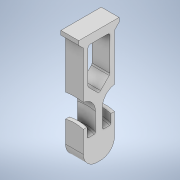
# Autodesk Inventor part: FS-04-SLBV1
Saved by Autodesk Inventor 2022 (Build 260153000, 153)
## iProperties
Created: 2022-01-12
Part Number: FS-04-SLBV1
Material: Generic
Document SubType Name: Modeling
Designer: Frank
Density: 1 g/cm^3
Appearance: Default
Author: Frank
Autodesk Inventor part; units mm, degrees
ref_plane "YZ Plane" through (0, 0, 0) normal (1, 0, 0) x (0, 1, 0)
ref_plane "XZ Plane" through (0, 0, 0) normal (0, 1, 0) x (-1, 0, 0)
ref_plane "XY Plane" through (0, 0, 0) normal (0, 0, 1) x (1, 0, 0)
sketch "Sketch1" plane through (0, 0, 0) normal (1, 0, 0) x (0, 1, 0)
  line L0 (0, 4.4) -> (0, -4.4)
  line L1 (0, -4.4) -> (-0.9, -4.4)
  line L2 (-0.9, -4.4) -> (-1.9, -3.4)
  line L3 (-1.9, -3.4) -> (-1.9, -3.4)
  line L4 (-1.9, -3.4) -> (-25, -3.4)
  line L5 (-25, -3.4) -> (-25, 3.4)
  line L6 (-25, 3.4) -> (-1.9, 3.4)
  line L7 (-1.9, 3.4) -> (-1.9, 3.4)
  line L8 (-1.9, 3.4) -> (-0.9, 4.4)
  line L9 (-0.9, 4.4) -> (0, 4.4)
  line L10 (0, 0) -> (-25, 0) construction
  line L11 (-24, 3.4) -> (-24, -3.4)
  line L12 (-12, 3.4) -> (-12, 0.75)
  line L13 (-12, 0.75) -> (-19, 0.75)
  line L14 (-19, 0.75) -> (-19, 2.6)
  line L15 (-19, 2.6) -> (-17, 2.6)
  line L16 (-17, 2.6) -> (-17, 3.4)
  line L17 (-12, -3.4) -> (-12, -0.75)
  line L18 (-12, -0.75) -> (-19, -0.75)
  line L19 (-19, -0.75) -> (-19, -2.6)
  line L20 (-19, -2.6) -> (-17, -2.6)
  line L21 (-17, -2.6) -> (-17, -3.4)
  dimension "d0" = 8.8
  dimension "d1" = 1.9
  dimension "d2" = 135
  dimension "d5" = 0.9
  dimension "d6" = 25
  dimension "d7" = 6.8
  dimension "d9" = 14
  dimension "d10" = 1
  dimension "d11" = 0.8
  dimension "d13" = 5
  dimension "d16" = 10
  dimension "d24" = 1.5
  constraints: 45 end point, 13 perpendicular, 6 point on line, 4 vertical, 2 midpoint, 2 parallel, 2 symmetric about line, 1 coincident, 1 horizontal, 6 other
  measures "d0" distance of L0.start L0.end
  measures "d1" distance between parallel lines of L0 L7
  measures "d2" angle of L7 L8
  measures "d5" distance of L0.start L8.end
  measures "d6" distance between parallel lines of L0 L5
  measures "d7" distance between parallel lines of L4 L6
  measures "d9" diameter of L16 L11
  measures "d10" distance of L5.end L11.start
  measures "d11" distance between parallel lines of L6 L15
  measures "d13" distance between parallel lines of L12 L16
  measures "d16" diameter of L14 L11
  measures "d24" distance between parallel lines of L18 L13
extrude "Extrusion1" add sketch "Sketch1" along normal mid plane 3.9
revolve "Revolution1" cut sketch "Sketch1" angle 360 about axis through (0, -24, 3.4) along (0, 0, -1) contours L12 L13 L14 L15 L16 L6 | L4 L21 L20 L19 L18 L17
fillet "Fillet1" radius 3 4 edges at (0, -12, 0.75) (0, -12, -0.75) (0, -25, -3.4) (0, -25, 3.4)
fillet "Fillet2" radius 0.3 4 edges at (0, -19, 2.6) (0, -19, 0.75) (0, -19, -0.75) (0, -19, -2.6)
sketch "Sketch2" plane through (1.95, 0, 0) normal (1, 0, 0) x (0, 0, -1)
  line L0 (-2.4, -1.9) -> (-2.4, -9.7595)
  line L1 (-2.4, -9.7595) -> (0, -12.1595)
  line L2 (0, -12.1595) -> (2.4, -9.7595)
  line L3 (2.4, -9.7595) -> (2.4, -1.9)
  line L4 (2.4, -1.9) -> (-2.4, -1.9)
  line L5 (-3.4, -1.9) -> (-3.4, -22) projected
  line L6 (0, 0) -> (0, -12.1595) construction
  line L7 (4.4, 0) -> (-4.4, 0) projected
  point P0 (-3.4, -12.1595)
  dimension "d19" = 1
  dimension "d20" = 135
  constraints: 12 end point, 2 horizontal alignment, 2 perpendicular, 1 parallel, 1 vertical, 2 other
  measures "d19" distance between parallel lines of L5 L0
  measures "d20" angle of L0 L1
extrude "Extrusion2" cut sketch "Sketch2" against normal through all
fillet "Fillet3" radius 0.5 5 edges at (0, -9.7595, 2.4) (0, -12.1595, 0) (0, -9.7595, -2.4) (0, -1.9, 2.4) (0, -1.9, -2.4)
body "Solid1"
